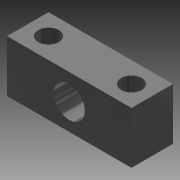
# Autodesk Inventor part: 8 ball arch mount
Saved by Autodesk Inventor 2012 (Build 160160000, 160)
## iProperties
Created: 2013-09-06
Part Number: 8 ball arch mount
Material: Default
Document SubType Name: Modeling
Designer: Bryce
Density: 1 g/cm^3
Author: Bryce
Autodesk Inventor part; units mm, degrees
ref_plane "YZ Plane" through (0, 0, 0) normal (1, 0, 0) x (0, 1, 0)
ref_plane "XZ Plane" through (0, 0, 0) normal (0, 1, 0) x (-1, 0, 0)
ref_plane "XY Plane" through (0, 0, 0) normal (0, 0, 1) x (1, 0, 0)
sketch "Sketch1" plane through (0, 0, 0) normal (0, 0, 1) x (1, 0, 0)
  line L0 (0, 0) -> (38.1, 0)
  line L1 (38.1, 0) -> (38.1, 15.875)
  line L2 (38.1, 15.875) -> (0, 15.875)
  line L3 (0, 15.875) -> (0, 0)
  circle A0 centre (19.05, 7.9375) radius 4.7625
  point P0 (0, 7.9375)
  point P1 (19.05, 15.875)
  dimension "d0" = 15.875
  dimension "d1" = 38.1
  dimension "d2" = 9.525
  dimension "d5" = 7.9375
  constraints: 8 end point, 2 midpoint, 2 parallel, 1 centre point, 1 horizontal, 1 perpendicular, 1 vertical alignment
  measures "d0" distance of L2.end L0.start
  measures "d1" distance of L0.start L0.end
  measures "d2" diameter of A0
  measures "d5" distance from line of L0 A0.centre
extrude "Extrusion1" add sketch "Sketch1" along normal blind 12.7
sketch "Sketch2" plane through (0, 15.875, 0) normal (0, 1, 0) x (1, 0, 0)
  line L0 (38.1, 0) -> (38.1, -12.7) projected
  line L1 (0, 0) -> (0, -12.7) projected
  circle A0 centre (6.35, -6.35) radius 3.175
  circle A1 centre (31.75, -6.35) radius 3.175
  point P0 (0, -6.35)
  dimension "d6" = 6.35
  dimension "d7" = 6.35
  dimension "d8" = 6.35
  dimension "d9" = 6.35
  constraints: 2 centre point, 2 horizontal alignment, 1 midpoint
  measures "d6" diameter of A0
  measures "d7" diameter of A1
  measures "d8" distance from line of L1 A0.centre
  measures "d9" distance from line of L0 A1.centre
extrude "Extrusion2" cut sketch "Sketch2" against normal blind 12.7
equation "\"d7\" = d6"
body "Solid1"
